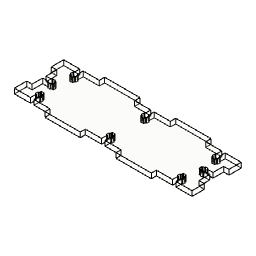
Carter_GD_KOSMOS3-0 (Autodesk Fusion 360 design; units mm, degrees)
Autodesk Fusion 360 part; units mm, degrees
note: some values were not read from the file. Set by a fixed rule: which sketch regions a step uses.
sketch "Esquisse1" plane through (0, 0, 0) normal (0, 0, 1) x (1, 0, 0)
  line L0 (-161.5, 274.6612) -> (-125.4, 274.6612)
  line L1 (-125.4, 274.6612) -> (-125.4, 280.0612)
  line L2 (-53.4, 280.0612) -> (-53.4, 274.6612)
  line L3 (-89.6, 274.6612) -> (-89.6, 280.0612)
  line L4 (18.5, 274.6612) -> (-17.6, 274.6612)
  line L5 (-17.6, 274.6612) -> (-17.6, 280.0612)
  line L6 (-125.4, 280.0612) -> (-89.6, 280.0612)
  line L7 (-53.4, 280.0612) -> (-17.6, 280.0612)
  line L8 (-194.564, 249.7112) -> (-161.5, 249.7112) construction
  line L9 (18.5, 249.7112) -> (43.7076, 249.7112) construction
  line L10 (-161.5, 224.7612) -> (-125.4, 224.7612)
  line L11 (-125.4, 224.7612) -> (-125.4, 219.3612)
  line L12 (-125.4, 219.3612) -> (-89.6, 219.3612)
  line L13 (-89.6, 224.7612) -> (-89.6, 219.3612)
  line L14 (-53.4, 224.7612) -> (-89.6, 224.7612)
  line L15 (-53.4, 219.3612) -> (-53.4, 224.7612)
  line L16 (-53.4, 219.3612) -> (-17.6, 219.3612)
  line L17 (-17.6, 224.7612) -> (-17.6, 219.3612)
  line L18 (18.5, 224.7612) -> (-17.6, 224.7612)
  line L19 (-17.6, 219.6612) -> (-53.4, 219.6612)
  line L20 (-89.6, 219.6612) -> (-125.4, 219.6612)
  line L21 (-161.5, 262.1862) -> (-156.1, 262.1862)
  line L22 (-156.1, 262.1862) -> (-156.1, 237.2362)
  line L23 (-156.1, 237.2362) -> (-161.5, 237.2362)
  line L24 (-161.5, 224.7612) -> (-161.5, 237.2362)
  line L25 (-161.5, 262.1862) -> (-161.5, 274.6612)
  line L26 (-71.5, 287.4578) -> (-71.5, 210) construction
  line L27 (18.5, 262.1862) -> (13.1, 262.1862)
  line L28 (13.1, 262.1862) -> (13.1, 237.2362)
  line L29 (13.1, 237.2362) -> (18.5, 237.2362)
  line L30 (18.5, 274.6612) -> (18.5, 262.1862)
  line L31 (18.5, 237.2362) -> (18.5, 224.7612)
  line L32 (-143.45, 274.6612) -> (-143.45, 267.0544) construction
  line L33 (-145.15, 274.6612) -> (-141.75, 274.6612)
  line L34 (-141.75, 274.6612) -> (-141.75, 268.6612)
  line L35 (-145.15, 268.6612) -> (-145.15, 274.6612)
  line L36 (-140.75, 268.6612) -> (-140.75, 265.9612)
  line L37 (-146.15, 265.9612) -> (-146.15, 268.6612)
  line L38 (-146.15, 268.6612) -> (-145.15, 268.6612)
  line L39 (-141.75, 268.6612) -> (-140.75, 268.6612)
  line L40 (-141.75, 265.9612) -> (-141.75, 264.4612)
  line L41 (-142.25, 263.9612) -> (-144.65, 263.9612)
  line L42 (-145.15, 264.4612) -> (-145.15, 265.9612)
  line L43 (-140.75, 265.9612) -> (-141.75, 265.9612)
  line L44 (-145.15, 265.9612) -> (-146.15, 265.9612)
  arc A0 (-145.15, 264.4612) -> (-144.65, 263.9612) centre (-144.65, 264.4612) ccw
  arc A1 (-142.25, 263.9612) -> (-141.75, 264.4612) centre (-142.25, 264.4612) ccw
  arc A2 (1.65, 263.9612) -> (2.15, 264.4612) centre (1.65, 264.4612) ccw
  line L45 (-0.75, 263.9612) -> (1.65, 263.9612)
  line L46 (2.15, 265.9612) -> (3.15, 265.9612)
  line L47 (-2.25, 265.9612) -> (-1.25, 265.9612)
  line L48 (2.15, 264.4612) -> (2.15, 265.9612)
  line L49 (-2.25, 268.6612) -> (-2.25, 265.9612)
  line L50 (0.45, 274.6612) -> (0.45, 267.0544) construction
  line L51 (3.15, 268.6612) -> (2.15, 268.6612)
  line L52 (-1.25, 265.9612) -> (-1.25, 264.4612)
  line L53 (-1.25, 268.6612) -> (-2.25, 268.6612)
  line L54 (2.15, 268.6612) -> (2.15, 274.6612)
  line L55 (3.15, 265.9612) -> (3.15, 268.6612)
  arc A3 (-1.25, 264.4612) -> (-0.75, 263.9612) centre (-0.75, 264.4612) ccw
  line L56 (-1.25, 274.6612) -> (-1.25, 268.6612)
  line L57 (-140.75, 233.4612) -> (-141.75, 233.4612)
  line L58 (-142.25, 235.4612) -> (-144.65, 235.4612)
  line L59 (-146.15, 233.4612) -> (-146.15, 230.7612)
  line L60 (-145.15, 234.9612) -> (-145.15, 233.4612)
  line L61 (-141.75, 230.7612) -> (-140.75, 230.7612)
  line L62 (-146.15, 230.7612) -> (-145.15, 230.7612)
  line L63 (-145.15, 233.4612) -> (-146.15, 233.4612)
  line L64 (-141.75, 233.4612) -> (-141.75, 234.9612)
  line L65 (-140.75, 230.7612) -> (-140.75, 233.4612)
  arc A4 (-141.75, 234.9612) -> (-142.25, 235.4612) centre (-142.25, 234.9612) ccw
  arc A5 (-144.65, 235.4612) -> (-145.15, 234.9612) centre (-144.65, 234.9612) ccw
  line L66 (-145.15, 230.7612) -> (-145.15, 224.7612)
  line L67 (-141.75, 224.7612) -> (-141.75, 230.7612)
  line L68 (3.15, 233.4612) -> (3.15, 230.7612)
  line L69 (-1.25, 233.4612) -> (-1.25, 234.9612)
  line L70 (3.15, 230.7612) -> (2.15, 230.7612)
  line L71 (-1.25, 230.7612) -> (-2.25, 230.7612)
  line L72 (2.15, 234.9612) -> (2.15, 233.4612)
  arc A6 (2.15, 234.9612) -> (1.65, 235.4612) centre (1.65, 234.9612) ccw
  line L73 (-0.75, 235.4612) -> (1.65, 235.4612)
  arc A7 (-0.75, 235.4612) -> (-1.25, 234.9612) centre (-0.75, 234.9612) ccw
  line L74 (2.15, 233.4612) -> (3.15, 233.4612)
  line L75 (-2.25, 230.7612) -> (-2.25, 233.4612)
  line L76 (-2.25, 233.4612) -> (-1.25, 233.4612)
  line L77 (-1.25, 224.7612) -> (-1.25, 230.7612)
  line L78 (2.15, 230.7612) -> (2.15, 224.7612)
  line L79 (-73.2, 274.6612) -> (-69.8, 274.6612)
  line L80 (-69.8, 274.6612) -> (-69.8, 268.6612)
  line L81 (-73.2, 268.6612) -> (-73.2, 274.6612)
  line L82 (-68.8, 265.9612) -> (-68.8, 268.6612)
  line L83 (-74.2, 268.6612) -> (-74.2, 265.9612)
  line L84 (-69.8, 265.9612) -> (-69.8, 264.4612)
  line L85 (-70.3, 263.9612) -> (-72.7, 263.9612)
  line L86 (-73.2, 264.4612) -> (-73.2, 265.9612)
  arc A8 (-70.3, 263.9612) -> (-69.8, 264.4612) centre (-70.3, 264.4612) ccw
  arc A9 (-73.2, 264.4612) -> (-72.7, 263.9612) centre (-72.7, 264.4612) ccw
  line L87 (-74.2, 265.9612) -> (-73.2, 265.9612)
  line L88 (-69.8, 265.9612) -> (-68.8, 265.9612)
  line L89 (-68.8, 268.6612) -> (-69.8, 268.6612)
  line L90 (-73.2, 268.6612) -> (-74.2, 268.6612)
  line L91 (-53.4, 274.6612) -> (-71.5, 274.6612)
  line L92 (-73.2, 274.6612) -> (-89.6, 274.6612)
  line L93 (-74.2, 233.4612) -> (-73.2, 233.4612)
  line L94 (-73.2, 234.9612) -> (-73.2, 233.4612)
  line L95 (-69.8, 233.4612) -> (-69.8, 234.9612)
  line L96 (-68.8, 233.4612) -> (-68.8, 230.7612)
  arc A10 (-72.7, 235.4612) -> (-73.2, 234.9612) centre (-72.7, 234.9612) ccw
  line L97 (-68.8, 230.7612) -> (-69.8, 230.7612)
  line L98 (-74.2, 230.7612) -> (-74.2, 233.4612)
  line L99 (-69.8, 233.4612) -> (-68.8, 233.4612)
  line L100 (-70.3, 235.4612) -> (-72.7, 235.4612)
  arc A11 (-69.8, 234.9612) -> (-70.3, 235.4612) centre (-70.3, 234.9612) ccw
  line L101 (-73.2, 230.7612) -> (-74.2, 230.7612)
  line L102 (-73.2, 230.7612) -> (-73.2, 224.7612)
  line L103 (-69.8, 224.7612) -> (-69.8, 230.7612)
  line L104 (-161.5, 249.7112) -> (43.7076, 249.7112) construction
  line L105 (-156.1, 248.0112) -> (-150.1, 248.0112)
  line L106 (-150.1, 251.4112) -> (-156.1, 251.4112)
  line L107 (-156.1, 251.4112) -> (-156.1, 248.0112)
  line L108 (-150.1, 252.4112) -> (-147.4, 252.4112)
  line L109 (-147.4, 247.0112) -> (-150.1, 247.0112)
  line L110 (-147.4, 251.2089) -> (-145.9, 251.2089)
  line L111 (-145.4, 250.7089) -> (-145.4, 248.3089)
  line L112 (-145.9, 247.8089) -> (-147.4, 247.8089)
  arc A12 (-145.9, 247.8089) -> (-145.4, 248.3089) centre (-145.9, 248.3089) ccw
  arc A13 (-145.4, 250.7089) -> (-145.9, 251.2089) centre (-145.9, 250.7089) ccw
  line L113 (-150.1, 247.0112) -> (-150.1, 248.0112)
  line L114 (-150.1, 251.4112) -> (-150.1, 252.4112)
  line L115 (-147.4, 252.4112) -> (-147.4, 251.2089)
  line L116 (-147.4, 247.8089) -> (-147.4, 247.0112)
  arc A14 (2.4, 248.3089) -> (2.9, 247.8089) centre (2.9, 248.3089) ccw
  line L117 (2.9, 247.8089) -> (4.4, 247.8089)
  line L118 (2.4, 250.7089) -> (2.4, 248.3089)
  line L119 (4.4, 247.8089) -> (4.4, 247.0112)
  line L120 (4.4, 251.2089) -> (2.9, 251.2089)
  line L121 (7.1, 252.4112) -> (4.4, 252.4112)
  line L122 (7.1, 251.4112) -> (7.1, 252.4112)
  line L123 (7.1, 247.0112) -> (7.1, 248.0112)
  arc A15 (2.9, 251.2089) -> (2.4, 250.7089) centre (2.9, 250.7089) ccw
  line L124 (4.4, 247.0112) -> (7.1, 247.0112)
  line L125 (4.4, 252.4112) -> (4.4, 251.2089)
  line L126 (7.1, 251.4112) -> (13.1, 251.4112)
  line L127 (13.1, 248.0112) -> (7.1, 248.0112)
  point P0 (-141.75, 263.9612)
  point P1 (-1.25, 263.9612)
  point P2 (-141.75, 235.4612)
  point P3 (-143.45, 232.3681)
  point P4 (-1.25, 235.4612)
  point P5 (0.45, 232.3681)
  point P6 (-69.8, 263.9612)
  point P7 (-73.2, 263.9612)
  point P8 (-73.2, 235.4612)
  point P9 (-69.8, 235.4612)
  point P10 (-145.4, 247.8089)
  point P11 (2.4, 247.8089)
  dimension "d84" = 5.4
  dimension "d85" = 5.4
  dimension "d86" = 5.4
  dimension "d87" = 35.8
  dimension "d88" = 36.1
  dimension "d89" = 36.2
  dimension "d90" = 35.8
  dimension "d91" = 36.1
  dimension "d93" = 60.4
  dimension "d94" = 5.4
  dimension "d95" = 24.95
  dimension "d96" = 49.9
  dimension "d97" = 12.475
  dimension "d98" = 90
  dimension "d99" = 18.05
  dimension "d101" = 3.4
  dimension "d102" = 1.7
  dimension "d103" = 6
  dimension "d104" = 5.4
  dimension "d105" = 2.7
  dimension "d106" = 2.7
  dimension "d107" = 3.4
  dimension "d108" = 1.7
  dimension "d109" = 2
  dimension "d110" = 0.5
  dimension "d111" = 3.4
  dimension "d112" = 1.7
  dimension "d113" = 6
  dimension "d114" = 2.7
  dimension "d115" = 5.4
  dimension "d116" = 2.7
  dimension "d117" = 3.4
  dimension "d118" = 1.7
  dimension "d119" = 2
  dimension "d120" = 0.5
  dimension "d121" = 3.4
  dimension "d122" = 1.7
  dimension "d123" = 6
  dimension "d124" = 2.7
  dimension "d125" = 5.4
  dimension "d126" = 2.7
  dimension "d127" = 3.4
  dimension "d128" = 2
  dimension "d129" = 0.5
  constraint horizontal L6
  constraint vertical L30
  constraint horizontal L19
  constraint vertical L24
  constraint horizontal L0
  constraint vertical L1
  constraint vertical L2
  constraint horizontal L91
  constraint vertical L3
  constraint horizontal L4
  constraint vertical L5
  constraint coincident L5.end L6
  constraint collinear L6 L7
  constraint perpendicular L8 L30
  constraint coincident L8.end L24
  constraint coincident L9.start L30
  constraint collinear L8 L9
  constraint symmetric L1.end L8 L11.end
  constraint symmetric L0.start L8 L10.start
  constraint symmetric L0.end L8 L10.end
  constraint symmetric L3.end L8 L12.end
  constraint symmetric L2.start L8 L15.start
  constraint symmetric L2.end L8 L14.start
  constraint symmetric L3.start L8 L13.start
  constraint symmetric L5.end L8 L16.end
  constraint symmetric L4.start L8 L18.start
  constraint symmetric L4.end L8 L17.start
  constraint coincident L11 L20.end
  constraint coincident L15 L19.end
  constraint coincident L13 L20.start
  constraint collinear L19 L20
  constraint coincident L17 L19.start
  constraint horizontal L21
  constraint vertical L22
  constraint horizontal L23
  constraint coincident L21.start L24
  constraint collinear L24 L25
  constraint perpendicular L14 L26
  constraint symmetric L21.start L26 L27.start
  constraint symmetric L21.end L26 L27.end
  constraint symmetric L22.end L26 L28.end
  constraint symmetric L23.end L26 L29.end
  constraint collinear L30 L31
  constraint coincident L0 L32.start
  constraint perpendicular L0 L32
  constraint horizontal L33
  constraint vertical L34
  constraint vertical L35
  constraint coincident L0 L33.start
  constraint horizontal L38
  constraint vertical L36
  constraint horizontal L43
  constraint vertical L37
  constraint collinear L38 L39
  constraint vertical L40
  constraint horizontal L41
  constraint vertical L42
  constraint coincident L42.end L43
  constraint collinear L43 L44
  constraint tangent L41 A0
  constraint tangent L42 A0
  constraint coincident P0 L40
  constraint coincident P0 L41
  constraint tangent L40 A1
  constraint tangent L41 A1
  constraint equal A0 A1
  constraint symmetric L26 L32.start L50.start
  constraint symmetric L26 L32.end L50.end
  constraint symmetric L26 L33.start L54.end
  constraint symmetric L26 L33.end L56.start
  constraint symmetric L26 L34.end L53.start
  constraint symmetric L26 L35.start L51.end
  constraint symmetric L26 L37.end L51.start
  constraint symmetric L26 L36.start L49.start
  constraint symmetric L26 L36.end L47.start
  constraint symmetric L26 L37.start L46.end
  constraint symmetric L26 L42.end L46.start
  constraint symmetric L26 L40.start L47.end
  constraint symmetric L26 P0 P1
  constraint symmetric L26 L41.end A2.start
  constraint symmetric L26 L42.start A2.end
  constraint symmetric L26 A0 A2
  constraint symmetric L26 L40.end L52.end
  constraint symmetric L26 L41.start L45.start
  constraint symmetric L26 A1 A3
  constraint symmetric L8 L32.end P3
  constraint symmetric L8 L33.start L66.end
  constraint symmetric L8 L33.end L67.start
  constraint symmetric L8 L34.end L61.start
  constraint symmetric L8 L35.start L62.end
  constraint symmetric L8 L37.end L59.end
  constraint symmetric L8 L36.start L61.end
  constraint symmetric L8 L36.end L57.start
  constraint symmetric L8 L37.start L59.start
  constraint symmetric L8 L42.end L60.end
  constraint symmetric L8 L40.start L57.end
  constraint symmetric L8 P0 P2
  constraint symmetric L8 L41.end L58.end
  constraint symmetric L8 L42.start L60.start
  constraint symmetric L8 A0 A5
  constraint symmetric L8 L40.end L64.end
  constraint symmetric L8 L41.start L58.start
  constraint symmetric L8 A1 A4
  constraint symmetric L8 L47.end L69.start
  constraint symmetric L8 P1 P4
  constraint symmetric L8 L47.start L75.end
  constraint symmetric L8 A2.end L72.start
  constraint symmetric L8 L52.end L69.end
  constraint symmetric L8 L53.start L71.start
  constraint symmetric L8 L51.start L68.end
  constraint symmetric L8 L51.end L70.end
  constraint symmetric L8 L49.start L71.end
  constraint symmetric L8 L45.start L73.start
  constraint symmetric L8 L46.start L72.end
  constraint symmetric L8 L50.end P5
  constraint symmetric L8 A2.start A6.end
  constraint symmetric L8 L46.end L68.start
  constraint symmetric L8 A2 A6
  constraint symmetric L8 L54.end L78.end
  constraint symmetric L8 A3 A7
  constraint symmetric L8 L56.start L77.start
  constraint horizontal L79
  constraint vertical L80
  constraint vertical L81
  constraint coincident L79.start L91
  constraint horizontal L87
  constraint vertical L82
  constraint horizontal L89
  constraint vertical L83
  constraint vertical L84
  constraint horizontal L85
  constraint vertical L86
  constraint coincident L81.start L89
  constraint coincident P6 L84
  constraint coincident P6 L85
  constraint tangent L84 A8
  constraint tangent L85 A8
  constraint coincident P7 L85
  constraint coincident P7 L86
  constraint tangent L85 A9
  constraint tangent L86 A9
  constraint equal A8 A9
  constraint collinear L87 L88
  constraint collinear L89 L90
  constraint coincident L26 L91.end
  constraint collinear L91 L92
  constraint symmetric L8 L79.start L102.end
  constraint symmetric L8 L79.end L103.start
  constraint symmetric L8 L80.end L97.end
  constraint symmetric L8 L81.start L101.start
  constraint symmetric L8 L83.end L93.start
  constraint symmetric L8 L82.start L96.start
  constraint symmetric L8 L82.end L96.end
  constraint symmetric L8 L83.start L98.start
  constraint symmetric L8 L86.end L93.end
  constraint symmetric L8 L84.start L95.start
  constraint symmetric L8 P6 P9
  constraint symmetric L8 P7 P8
  constraint symmetric L8 L84.end L95.end
  constraint symmetric L8 L85.start L100.start
  constraint symmetric L8 A8 A11
  constraint symmetric L8 L85.end A10.start
  constraint symmetric L8 L86.start L94.start
  constraint symmetric L8 A9 A10
  constraint horizontal L105
  constraint horizontal L106
  constraint vertical L107
  constraint coincident L22 L105.start
  constraint horizontal L108
  constraint vertical L115
  constraint horizontal L109
  constraint vertical L113
  constraint horizontal L110
  constraint vertical L111
  constraint horizontal L112
  constraint coincident P10 L111
  constraint coincident P10 L112
  constraint tangent L111 A12
  constraint tangent L112 A12
  constraint tangent L110 A13
  constraint tangent L111 A13
  constraint equal A12 A13
  constraint collinear L113 L114
  constraint collinear L115 L116
  constraint symmetric L26 L105.start L127.start
  constraint symmetric L26 L105.end L123.end
  constraint symmetric L26 L106.start L122.start
  constraint symmetric L26 L106.end L126.end
  constraint symmetric L26 L108.start L121.start
  constraint symmetric L26 L108.end L121.end
  constraint symmetric L26 L109.start L119.end
  constraint symmetric L26 L109.end L123.start
  constraint symmetric L26 L110.start L120.start
  constraint symmetric L26 P10 P11
  constraint symmetric L26 L112.end L117.end
  constraint symmetric L26 L111.end A14.start
  constraint symmetric L26 L112.start A14.end
  constraint symmetric L26 A12 A14
  constraint symmetric L26 L110.end L120.end
  constraint symmetric L26 L111.start L118.start
  constraint symmetric L26 A13 A15
  measures "d84" distance of L1.end L0.end
  measures "d85" distance of L3.end L3.start
  measures "d86" distance of L5.end L4.end
  measures "d87" distance of L1.end L3.end
  measures "d88" distance of L0.start L0.end
  measures "d89" distance of L2.end L3.start
  measures "d90" distance of L2.start L5.end
  measures "d91" distance of L4.start L4.end
  measures "d93" distance of L6 L19
  measures "d94" distance of L21.start L21.end
  measures "d95" distance of L21.end L22.end
  measures "d96" distance of L0.start L10.start
  measures "d97" distance of L8 L21
  measures "d98" distance of L25 L26
  measures "d99" distance of L25 L32
  measures "d101" distance of L33.start L33.end
  measures "d102" distance of L32 L35
  measures "d103" distance of L33.start L35.start
  measures "d104" distance of L37.end L36.start
  measures "d105" distance of L32 L36
  measures "d106" distance of L37.end L37.start
  measures "d107" distance of L40 L42
  measures "d108" distance of L32 L40
  measures "d109" distance of L40.start P0
  measures "d110" radius of A0
  measures "d111" distance of L80 L81
  measures "d112" distance of L26 L80
  measures "d113" distance of L79.start L81.start
  measures "d114" distance of L83.end L83.start
  measures "d115" distance of L82 L83
  measures "d116" distance of L26 L83
  measures "d117" distance of P6 P7
  measures "d118" distance of L26 L84
  measures "d119" distance of L84.start P6
  measures "d120" radius of A8
  measures "d121" distance of L105.start L106.end
  measures "d122" distance of L104 L105
  measures "d123" distance of L106.start L106.end
  measures "d124" distance of L108.start L108.end
  measures "d125" distance of L108 L109
  measures "d126" distance of L104 L109
  measures "d127" distance of L110.start L112.end
  measures "d128" distance of P10 L112.end
  measures "d129" radius of A12
extrude "Extrusion1" add sketch "Esquisse1" along normal blind 5 contours L0 L1 L2 L3 L4 L5 L6 L7 L10 L11 L13 L14 L15 L17 L18 L19 L20 L21 L22 L23 L24 L25 L27 L28 L29 L30 L31 L34 L35 L36 L37 L38 L39 L40 L41 L42 L43 L44 A0 A1 A2 L45 L46 L47 L48 L49 L51 L52 L53 L54 L55 A3 L56 L57 L58 L59 L60 L61 L62 L63 L64 L65 A4 A5 L66 L67 L68 L69 L70 L71 L72 A6 L73 A7 L74 L75 L76 L77 L78 L80 L81 L82 L83 L84 L85 L86 A8 A9 L87 L88 L89 L90 L91 L92 L93 L94 L95 L96 A10 L97 L98 L99 L100 A11 L101 L102 L103 L105 L106 L108 L109 L110 L111 L112 A12 A13 L113 L114 L115 L116 A14 L117 L118 L119 L120 L121 L122 L123 A15 L124 L125 L126 L127
equation "d84 = 5.3 mm + 0.1 mm"
equation "d85 = d84"
equation "d86 = d84"
equation "d87 = 36 mm - 0.2 mm"
equation "d88 = 36 mm + 0.1 mm"
equation "d89 = 36 mm + 0.2 mm"
equation "d90 = d87"
equation "d91 = d88"
equation "d94 = d84"
equation "d95 = d96 / 2"
equation "d97 = d95 / 2"
equation "d98 = ( 180 / 2 ) * 1 mm"
equation "d99 = d88 / 2"
equation "d102 = d101 / 2"
equation "d105 = d104 / 2"
equation "d107 = d101"
equation "d108 = d107 / 2"
equation "d111 = d101"
equation "d112 = d111 / 2"
equation "d113 = d103"
equation "d114 = d106"
equation "d115 = d104"
equation "d116 = d115 / 2"
equation "d117 = d111"
equation "d118 = d117 / 2"
equation "d119 = d109"
equation "d121 = d101"
equation "d122 = d121 / 2"
equation "d123 = d103"
equation "d124 = d106"
equation "d125 = d104"
equation "d126 = d125 / 2"
equation "d127 = d121"
equation "d128 = d109"
